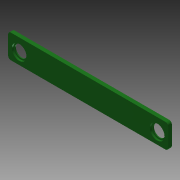
# Autodesk Inventor part: arm1a
Saved by Autodesk Inventor 2013 (Build 170138000, 138)
## iProperties
Created: 2014-06-28
Part Number: arm1a
Material: Generic
Document SubType Name: Modeling
Designer: Masta
Density: 1 g/cm^3
Author: Masta
Autodesk Inventor part; units mm, degrees
ref_plane "YZ Plane" through (0, 0, 0) normal (1, 0, 0) x (0, 1, 0)
ref_plane "XZ Plane" through (0, 0, 0) normal (0, 1, 0) x (-1, 0, 0)
ref_plane "XY Plane" through (0, 0, 0) normal (0, 0, 1) x (1, 0, 0)
sketch "Sketch1" plane through (0, 0, 0) normal (0, 1, 0) x (-1, 0, 0)
  line L0 (172, 20) -> (172, 0)
  line L1 (2, 20) -> (2, 0)
  line L2 (43, 20) -> (43, 0)
  line L3 (131, 20) -> (131, 0)
  line L4 (129, 20) -> (129, 0)
  line L5 (174, 24) -> (174, 0)
  line L6 (45, 20) -> (45, 0)
  line L7 (0, 24) -> (0, 0)
  line L8 (0, 0) -> (174, 0)
  line L9 (0, 24) -> (174, 24)
  line L10 (131, 20) -> (172, 20)
  line L11 (2, 20) -> (43, 20)
  line L12 (45, 20) -> (129, 20)
  line L13 (0, 0) -> (174, 0)
  line L14 (174, 0) -> (174, -2)
  line L15 (174, -2) -> (0, -2)
  line L16 (0, -2) -> (0, 0)
  line L17 (2, 10) -> (172, 10) construction
  line L18 (162, 20) -> (162, 0) construction
  line L19 (12, 20) -> (12, 0) construction
  circle A0 centre (12, 10) radius 8
  circle A1 centre (12, 10) radius 6.5
  circle A2 centre (162, 10) radius 6.5
  circle A3 centre (162, 10) radius 8
  dimension "d4" = 41
  dimension "d5" = 41
  dimension "d7" = 2
  dimension "d8" = 2
  dimension "d9" = 2
  dimension "d10" = 2
  dimension "d12" = 174
  dimension "d17" = 4
  dimension "d20" = 20
  dimension "d21" = 2
  dimension "d22" = 10
  dimension "d23" = 10
  dimension "d24" = 16
  dimension "d25" = 13
  constraints: 40 end point, 10 point on line, 7 perpendicular, 4 centre point, 4 midpoint, 3 coincident, 3 collinear, 3 parallel, 2 equal radius, 2 horizontal
  measures "d4" distance between parallel lines of L2 L1
  measures "d5" distance between parallel lines of L0 L3
  measures "d7" distance between parallel lines of L1 L7
  measures "d8" distance between parallel lines of L2 L6
  measures "d9" distance between parallel lines of L3 L4
  measures "d10" distance between parallel lines of L0 L5
  measures "d12" distance of L7.start L5.start
  measures "d17" distance between parallel lines of L9 L11
  measures "d20" distance between parallel lines of L8 L10
  measures "d21" distance of L13.end L14.end
  measures "d22" distance between parallel lines of L1 L19
  measures "d23" distance between parallel lines of L0 L18
  measures "d24" diameter of A0
  measures "d25" diameter of A1
extrude "Extrusion1" add sketch "Sketch1" against normal blind 3 contours L10 L3 L8 L4 L12 L6 L2 L11 L1 L7 L9 L5 L0 | L0 L8 L3 L10 | L8 L14 L15 L16 | L8 L6 L12 L4 | L8 L1 L11 L2
extrude "Extrusion2" add sketch "Sketch1" along normal blind 1 contours L10 L3 L8 L4 L12 L6 L2 L11 L1 L7 L9 L5 L0 | L8 L14 L15 L16
extrude "Extrusion3" add sketch "Sketch1" against normal blind 1 contours A0 | A3
fillet "Fillet1" radius 3 4 edges at (-174, -1, -2) (-174, -1, 24) (0, -1, 24) (0, -1, -2)
body "Solid1"
